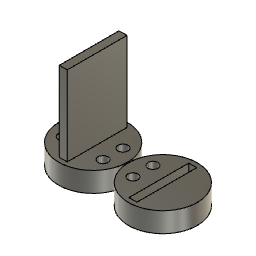
flightcomputerholder v0 (Autodesk Fusion 360 design; units mm, degrees)
Autodesk Fusion 360 part; units mm, degrees
sketch "Sketch1" plane through (0, 0, 0) normal (0, 0, 1) x (1, 0, 0)
  circle A0 centre (0, 0) radius 34.5
  dimension "d1" = 69
  constraint coincident A0.centre origin
  measures "d1" diameter of A0
extrude "Extrude1" add sketch "Sketch1" along normal blind 20 makes body 1
sketch "Sketch2" plane through (0, 0, 20) normal (0, 0, 1) x (-1, 0, 0)
  circle A0 centre (0, 0) radius 34.5
  line L0 (0, 0) -> (-4, 0)
  line L1 (0, 0) -> (4, 0)
  line L2 (4, 0) -> (-4, 0)
  line L3 (-4, 0) -> (-4, -30)
  line L4 (-4, -30) -> (4, -30)
  line L5 (4, -30) -> (4, 0)
  line L6 (4, 0) -> (-4, 0)
  line L7 (-4, 0) -> (-4, 30)
  line L8 (-4, 30) -> (4, 30)
  line L9 (4, 30) -> (4, 0)
  dimension "d4" = 4
  dimension "d5" = 4
  constraint coincident A0.centre L0.start
  constraint horizontal L0
  constraint parallel L0 L1
  constraint horizontal L2
  constraint vertical L3
  constraint horizontal L4
  constraint vertical L5
  constraint horizontal L6
  constraint vertical L7
  constraint horizontal L8
  constraint vertical L9
  measures "d4" distance of A0.centre L0.end
  measures "d5" distance of A0.centre L1.end
extrude "Extrude2" add sketch "Sketch2" along normal blind 80 contours L0 L1 L2 L3 L4 L5 L6 | L0 L1 L2 L6 L7 L8 L9 bodies 1
sketch "Sketch3" plane through (0, 0, 20) normal (0, 0, 1) x (-1, 0, 0)
  line L0 (-4, 30) -> (4, 30)
  line L1 (4, 30) -> (4, -30)
  line L2 (4, -30) -> (-4, -30)
  line L3 (-4, -30) -> (-4, 30)
  circle A0 centre (0, 0) radius 34.5
  circle A1 centre (20, -10) radius 5
  circle A2 centre (-20, 10) radius 5
  circle A3 centre (20, 10) radius 5
  circle A4 centre (-20, -10) radius 5
  dimension "d8" = 10
  dimension "d9" = 10
  dimension "d10" = 10
  dimension "d11" = 10
  measures "d8" diameter of A1
  measures "d9" diameter of A2
  measures "d10" diameter of A3
  measures "d11" diameter of A4
extrude "Extrude3" cut sketch "Sketch3" against normal blind 20 contours A1 | A2 | A3 | A4 bodies 1
move_body "Move1" bodies 1 to x (1, 0, 0) y (0, 1, 0) z (0, 0, 1) at (-80, 0, 0)
sketch "Sketch4" plane through (0, 0, 0) normal (0, 0, 1) x (1, 0, 0)
  circle A0 centre (0, 0) radius 34.5
  dimension "d14" = 69
  constraint coincident A0.centre origin
  measures "d14" diameter of A0
extrude "Extrude4" add sketch "Sketch4" along normal blind 20 separate body makes body 2
sketch "Sketch5" plane through (0, 0, 20) normal (0, 0, 1) x (-1, 0, 0)
  circle A0 centre (0, 0) radius 34.5
  line L0 (0, 0) -> (-4, 0)
  line L1 (0, 0) -> (4, 0)
  line L2 (4, 0) -> (-4, 0)
  line L3 (-4, 0) -> (-4, -30)
  line L4 (-4, -30) -> (4, -30)
  line L5 (4, -30) -> (4, 0)
  line L6 (-4, 0) -> (4, 0)
  line L7 (4, 0) -> (4, 30)
  line L8 (4, 30) -> (-4, 30)
  line L9 (-4, 30) -> (-4, 0)
  dimension "d17" = 4
  dimension "d18" = 4
  dimension "d19" = 8
  dimension "d20" = 30
  dimension "d21" = 8
  dimension "d22" = 30
  constraint coincident A0.centre L0.start
  constraint horizontal L0
  constraint parallel L0 L1
  constraint horizontal L2
  constraint vertical L3
  constraint horizontal L4
  constraint vertical L5
  constraint horizontal L6
  constraint vertical L7
  constraint horizontal L8
  constraint vertical L9
  measures "d17" distance of A0.centre L0.end
  measures "d18" distance of A0.centre L1.end
  measures "d19" distance of L1.end L0.end
  measures "d20" distance of L1.end L4.end
  measures "d21" distance of L0.end L1.end
  measures "d22" distance of L0.end L8.end
extrude "Extrude5" cut sketch "Sketch5" against normal blind 8 contours L0 L1 L2 L3 L4 L5 L6 | L0 L1 L2 L6 L7 L8 L9 bodies 2
sketch "Sketch6" plane through (0, 0, 20) normal (0, 0, 1) x (-1, 0, 0)
  line L0 (4, -30) -> (-4, -30)
  line L1 (-4, -30) -> (-4, 30)
  line L2 (-4, 30) -> (4, 30)
  line L3 (4, 30) -> (4, -30)
  circle A0 centre (0, 0) radius 34.5
  circle A1 centre (20, -10) radius 5
  circle A2 centre (20, 10) radius 5
  dimension "d25" = 10
  dimension "d26" = 10
  measures "d25" diameter of A1
  measures "d26" diameter of A2
extrude "Extrude6" cut sketch "Sketch6" against normal blind 20 contours A1 | A2 bodies 2
move_body "Move2" bodies 2 1 to x (1, 0, 0) y (0, 1, 0) z (0, 0, 1) at (40, 0, 0)
move_body "Move3" bodies 2 to x (1, 0, 0) y (0, 1, 0) z (0, 0, 1) at (-10, 0, 0)
move_body "Move4" bodies 2 1 to x (1, 0, 0) y (0, 1, 0) z (0, 0, 1) at (5, 0, 0)
